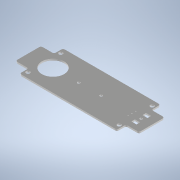
# Autodesk Inventor part: Interstage B2
Saved by Autodesk Inventor 2020.3 (Build 243373000, 373)
## iProperties
Created: 2020-05-18
Part Number: Interstage B2
Material: Genérico
Document SubType Name: Modeling
Designer: javic
Density: 1 g/cm^3
Appearance: Valor por defecto
Author: javic
Autodesk Inventor part; units mm, degrees
ref_plane "YZ Plane" through (0, 0, 0) normal (1, 0, 0) x (0, 1, 0)
ref_plane "XZ Plane" through (0, 0, 0) normal (0, 1, 0) x (-1, 0, 0)
ref_plane "XY Plane" through (0, 0, 0) normal (0, 0, 1) x (1, 0, 0)
sketch "Boceto1" plane through (0, 0, 0) normal (0, 1, 0) x (-1, 0, 0)
  arc A0 (-10.02, 7.27) -> (-8.75, 6) centre (-8.75, 7.27) ccw
  line L0 (-8.75, 6) -> (-2.54, 6)
  arc A1 (-1.27, 4.73) -> (-2.54, 6) centre (-2.54, 4.73) ccw
  line L1 (-1.27, 4.73) -> (-1.27, 1.27)
  arc A2 (-1.27, 1.27) -> (0, 0) centre (0, 1.27) ccw
  line L2 (0, 0) -> (62.46, 0)
  arc A3 (62.46, 0) -> (63.73, 1.27) centre (62.46, 1.27) ccw
  line L3 (63.73, 1.27) -> (63.73, 4.73)
  arc A4 (65, 6) -> (63.73, 4.73) centre (65, 4.73) ccw
  line L4 (65, 6) -> (71.21, 6)
  arc A5 (71.21, 6) -> (72.48, 7.27) centre (71.21, 7.27) ccw
  line L5 (72.48, 7.27) -> (72.48, 21.73)
  arc A6 (72.48, 21.73) -> (71.21, 23) centre (71.21, 21.73) ccw
  line L6 (71.21, 23) -> (65, 23)
  arc A7 (63.73, 24.27) -> (65, 23) centre (65, 24.27) ccw
  line L7 (63.73, 24.27) -> (63.73, 27.73)
  arc A8 (63.73, 27.73) -> (62.46, 29) centre (62.46, 27.73) ccw
  line L8 (62.46, 29) -> (0, 29)
  arc A9 (0, 29) -> (-1.27, 27.73) centre (0, 27.73) ccw
  line L9 (-1.27, 27.73) -> (-1.27, 24.27)
  arc A10 (-2.54, 23) -> (-1.27, 24.27) centre (-2.54, 24.27) ccw
  line L10 (-2.54, 23) -> (-8.75, 23)
  arc A11 (-8.75, 23) -> (-10.02, 21.73) centre (-8.75, 21.73) ccw
  line L11 (-10.02, 21.73) -> (-10.02, 7.27)
  circle A12 centre (55.955, 14.5) radius 7.4
  circle A13 centre (61.755, 25.475) radius 1.25
  circle A14 centre (0.755, 3.475) radius 1.25
  circle A15 centre (0.755, 25.475) radius 1.25
  circle A16 centre (61.755, 3.475) radius 1.25
  circle A17 centre (38.73, 14.5) radius 0.9
  circle A18 centre (23.73, 14.5) radius 0.9
  point P0 (0, 0)
  constraints: 27 tangent, 24 end point, 24 point on circle, 19 centre point, 15 equal radius, 4 parallel, 4 perpendicular
extrude "Extrusión1" add sketch "Boceto1" along normal blind 1.04
sketch "Boceto2" plane through (0, 1.04, 0) normal (0, 1, 0) x (1, 0, 0)
  circle A0 centre (3.02, -14.5) radius 0.9
  line L0 (-71.21, -23) -> (-65, -23) projected
  line L1 (-72.48, -7.27) -> (-72.48, -21.73) projected
  line L2 (2.54, -23) -> (8.75, -23) projected
  line L3 (10.02, -21.73) -> (10.02, -7.27) projected
  point P0 (0, 0)
  dimension "d3" = 1.8
  dimension "d6" = 8.5
  dimension "d7" = 7
  constraints: 1 centre point
  measures "d3" diameter of A0
  measures "d6" distance from line of L2 A0.centre
  measures "d7" distance from line of L3 A0.centre
hole "Agujero1" at (3.02, 1.04, 14.5) direction (0, -1, 0) diameter 1.8 end through all
sketch "Boceto3" plane through (0, 0, 0) normal (0, -1, 0) x (1, 0, 0)
  circle A0 centre (-3.08, 17.04) radius 0.4
  line L0 (10.02, 21.73) -> (10.02, 7.27) projected
  line L1 (-62.46, 29) -> (0, 29) projected
  circle A1 centre (-3.08, 14.5) radius 0.4
  circle A2 centre (-3.08, 11.96) radius 0.4
  line L2 (0, 0) -> (-62.46, 0) projected
  dimension "d15" = 0.8
  dimension "d16" = 13.1
  dimension "d17" = 11.96
  dimension "d18" = 0.8
  dimension "d19" = 0.8
  dimension "d20" = 13.1
  dimension "d21" = 13.1
  dimension "d22" = 11.96
  dimension "d23" = 2.54
  dimension "d24" = 2.54
  constraints: 3 centre point
  measures "d15" diameter of A0
  measures "d16" distance from line of L0 A0.centre
  measures "d17" distance from line of L1 A0.centre
  measures "d18" diameter of A1
  measures "d19" diameter of A2
  measures "d20" distance from line of A1.centre L0
  measures "d21" distance from line of A2.centre L0
  measures "d22" distance from line of L2 A2.centre
  measures "d23" distance of A2.centre A1.centre
  measures "d24" distance of A1.centre A0.centre
hole "Agujero2" at (-3.08, 0, 17.04) at (-3.08, 0, 14.5) at (-3.08, 0, 11.96) direction (0, 1, 0) diameter 0.8 end through all
sketch "Boceto4" plane through (0, 1.04, 0) normal (0, 1, 0) x (1, 0, 0)
  line L0 (4.72, -19.4) -> (1.32, -19.4)
  line L1 (1.32, -19.4) -> (1.32, -17)
  line L2 (1.32, -17) -> (4.72, -17)
  line L3 (4.72, -17) -> (4.72, -19.4)
  line L4 (2.54, -23) -> (8.75, -23) projected
  line L5 (10.02, -21.73) -> (10.02, -7.27) projected
  line L6 (4.72, -12) -> (1.32, -12)
  line L7 (1.32, -12) -> (1.32, -9.6)
  line L8 (1.32, -9.6) -> (4.72, -9.6)
  line L9 (4.72, -9.6) -> (4.72, -12)
  line L10 (8.75, -6) -> (2.54, -6) projected
  point P0 (0, 0)
  dimension "d32" = 3.4
  dimension "d33" = 2.4
  dimension "d34" = 3.6
  dimension "d35" = 5.3
  dimension "d36" = 2.4
  dimension "d37" = 5.3
  dimension "d38" = 3.6
  constraints: 16 end point, 4 parallel, 2 horizontal, 2 perpendicular
  measures "d32" distance of L1.end L2.end
  measures "d33" distance of L0.end L1.end
  measures "d34" distance between parallel lines of L4 L0
  measures "d35" distance between parallel lines of L5 L3
  measures "d36" distance of L6.end L7.end
  measures "d37" distance between parallel lines of L5 L9
  measures "d38" distance between parallel lines of L10 L8
extrude "Extrusión2" cut sketch "Boceto4" against normal through all
